Autodesk Fusion 360 part; units mm, degrees
(part 2 of 2)
sketch "Skizze17" plane through (0, 8, 0) normal (0, 1, 0) x (-1, 0, 0)
  spline S0 degree 3 poles (13.6382, 4.4313) (13.5302, 4.764) (13.3982, 5.084) (13.1091, 5.6313) (12.979, 5.7983) (12.7664, 6.018) (12.6585, 6.0998) (12.4173, 6.2178) (12.2929, 6.2453) (11.9322, 6.267) (11.6792, 6.209) (10.9713, 5.9696) (10.4381, 5.7266) (9.6899, 5.336) (9.4122, 5.1477) (9.0348, 4.7941) (8.8234, 4.5529) (8.5425, 3.9264) (8.498, 3.6504) (8.4775, 3.1972) (8.4959, 2.9778) (8.559, 2.7826) (8.5803, 2.717) (8.6261, 2.5931) (8.8115, 2.2891) (8.9377, 2.1162) (9.2854, 1.782) (9.4864, 1.6516) (10.0239, 1.4143) (10.3245, 1.381) (10.6864, 1.3735) (11.2116, 1.3812) (12.7231, 1.7144) (12.9818, 1.813) (13.2963, 1.9497) (13.4267, 2.0277) (13.6341, 2.2058) (13.7097, 2.3032) (13.8353, 2.5437) (13.8748, 2.6944) (13.921, 3.1631) (13.8758, 3.4676) (13.7815, 3.9466) (13.7161, 4.1922) (13.6382, 4.4313) knots -0.557189 -0.557189 -0.557189 -0.557189 -0.528825 -0.528825 -0.49746 -0.49746 -0.469449 -0.469449 -0.438886 -0.438886 -0.380684 -0.380684 -0.293014 -0.293014 -0.196609 -0.196609 -0.126355 -0.126355 -0.061556 -0.061556 0 0 0 0.020699 0.020699 0.037386 0.037386 0.056379 0.056379 0.086419 0.086419 0.099545 0.099545 0.108574 0.108574 0.118089 0.118089 0.127425 0.127425 0.139171 0.139171 0.160415 0.160415 0.180805 0.180805 0.180805 0.180805
  spline S1 degree 3 poles (8.4288, 11.6013) (8.146, 11.8071) (7.8511, 11.9884) (7.2955, 12.2611) (7.0921, 12.3198) (6.791, 12.3725) (6.6556, 12.3753) (6.391, 12.329) (6.2743, 12.2782) (5.9697, 12.0837) (5.7991, 11.8881) (5.3671, 11.2782) (5.0786, 10.7683) (4.7028, 10.0125) (4.5889, 9.6969) (4.4914, 9.189) (4.4621, 8.8696) (4.6031, 8.1977) (4.7294, 7.9482) (4.9792, 7.5696) (5.123, 7.4029) (5.2888, 7.2821) (5.3446, 7.2414) (5.4545, 7.1681) (5.7831, 7.0312) (5.9869, 6.9655) (6.4647, 6.8995) (6.7039, 6.9122) (7.2782, 7.0361) (7.5409, 7.1858) (7.8381, 7.3925) (8.2585, 7.7074) (9.2855, 8.8654) (9.4368, 9.0973) (9.6109, 9.3927) (9.6706, 9.5325) (9.7337, 9.7985) (9.7376, 9.9217) (9.6979, 10.1901) (9.6412, 10.3352) (9.4031, 10.7416) (9.1875, 10.9614) (8.8297, 11.2934) (8.6324, 11.4537) (8.4288, 11.6013) knots -0.557189 -0.557189 -0.557189 -0.557189 -0.528825 -0.528825 -0.49746 -0.49746 -0.469449 -0.469449 -0.438886 -0.438886 -0.380684 -0.380684 -0.293014 -0.293014 -0.196609 -0.196609 -0.126355 -0.126355 -0.061556 -0.061556 0 0 0 0.020699 0.020699 0.037386 0.037386 0.056379 0.056379 0.086419 0.086419 0.099545 0.099545 0.108574 0.108574 0.118089 0.118089 0.127425 0.127425 0.139171 0.139171 0.160415 0.160415 0.180805 0.180805 0.180805 0.180805
  spline S2 degree 3 poles (-13.6382, -4.4313) (-13.5302, -4.764) (-13.3982, -5.084) (-13.1091, -5.6313) (-12.979, -5.7983) (-12.7664, -6.018) (-12.6585, -6.0998) (-12.4173, -6.2178) (-12.2929, -6.2453) (-11.9322, -6.267) (-11.6792, -6.209) (-10.9713, -5.9696) (-10.4381, -5.7266) (-9.6899, -5.336) (-9.4122, -5.1477) (-9.0348, -4.7941) (-8.8234, -4.5529) (-8.5425, -3.9264) (-8.498, -3.6504) (-8.4775, -3.1972) (-8.4959, -2.9778) (-8.559, -2.7826) (-8.5803, -2.717) (-8.6261, -2.5931) (-8.8115, -2.2891) (-8.9377, -2.1162) (-9.2854, -1.782) (-9.4864, -1.6516) (-10.0239, -1.4143) (-10.3245, -1.381) (-10.6864, -1.3735) (-11.2116, -1.3812) (-12.7231, -1.7144) (-12.9818, -1.813) (-13.2963, -1.9497) (-13.4267, -2.0277) (-13.6341, -2.2058) (-13.7097, -2.3032) (-13.8353, -2.5437) (-13.8748, -2.6944) (-13.921, -3.1631) (-13.8758, -3.4676) (-13.7815, -3.9466) (-13.7161, -4.1922) (-13.6382, -4.4313) knots -0.557189 -0.557189 -0.557189 -0.557189 -0.528825 -0.528825 -0.49746 -0.49746 -0.469449 -0.469449 -0.438886 -0.438886 -0.380684 -0.380684 -0.293014 -0.293014 -0.196609 -0.196609 -0.126355 -0.126355 -0.061556 -0.061556 0 0 0 0.020699 0.020699 0.037386 0.037386 0.056379 0.056379 0.086419 0.086419 0.099545 0.099545 0.108574 0.108574 0.118089 0.118089 0.127425 0.127425 0.139171 0.139171 0.160415 0.160415 0.180805 0.180805 0.180805 0.180805
  spline S3 degree 3 poles (13.6382, -4.4313) (13.7464, -4.0987) (13.8277, -3.7622) (13.9155, -3.1495) (13.9084, -2.9379) (13.8655, -2.6353) (13.8263, -2.5057) (13.7005, -2.2684) (13.6161, -2.173) (13.337, -1.9434) (13.0982, -1.8416) (12.3848, -1.6193) (11.8106, -1.5025) (10.9757, -1.3786) (10.6404, -1.3678) (10.1272, -1.432) (9.8143, -1.5029) (9.2189, -1.8446) (9.0206, -2.0418) (8.7377, -2.3964) (8.6236, -2.5846) (8.56, -2.7797) (8.5386, -2.8453) (8.5028, -2.9724) (8.4741, -3.3273) (8.4746, -3.5414) (8.5595, -4.0162) (8.6455, -4.2398) (8.9408, -4.7477) (9.1644, -4.9513) (9.4528, -5.1701) (9.8822, -5.4726) (11.3009, -6.0915) (11.5681, -6.1637) (11.9029, -6.238) (12.0543, -6.2516) (12.3268, -6.2294) (12.4451, -6.195) (12.6881, -6.0743) (12.8087, -5.9756) (13.1216, -5.6236) (13.264, -5.3506) (13.4692, -4.9077) (13.5607, -4.6705) (13.6382, -4.4313) knots -0.557189 -0.557189 -0.557189 -0.557189 -0.528825 -0.528825 -0.49746 -0.49746 -0.469449 -0.469449 -0.438886 -0.438886 -0.380684 -0.380684 -0.293014 -0.293014 -0.196609 -0.196609 -0.126355 -0.126355 -0.061556 -0.061556 0 0 0 0.020699 0.020699 0.037386 0.037386 0.056379 0.056379 0.086419 0.086419 0.099545 0.099545 0.108574 0.108574 0.118089 0.118089 0.127425 0.127425 0.139171 0.139171 0.160415 0.160415 0.180805 0.180805 0.180805 0.180805
  spline S4 degree 3 poles (8.4288, -11.6013) (8.7119, -11.3959) (8.9755, -11.1714) (9.4066, -10.7273) (9.5253, -10.552) (9.6685, -10.2819) (9.7129, -10.154) (9.7506, -9.8881) (9.7384, -9.7613) (9.6475, -9.4116) (9.5142, -9.1888) (9.0677, -8.5896) (8.6718, -8.1576) (8.0692, -7.5667) (7.8043, -7.3609) (7.3514, -7.1111) (7.0566, -6.9846) (6.374, -6.9111) (6.0977, -6.954) (5.6604, -7.0746) (5.4575, -7.1598) (5.2913, -7.2802) (5.2354, -7.3207) (5.1318, -7.4026) (4.9, -7.6728) (4.7745, -7.8463) (4.5641, -8.2803) (4.5023, -8.5117) (4.4427, -9.0962) (4.5039, -9.3924) (4.6086, -9.7389) (4.7781, -10.2361) (5.5621, -11.5706) (5.7359, -11.7861) (5.963, -12.043) (6.0775, -12.143) (6.311, -12.2852) (6.427, -12.327) (6.6945, -12.3721) (6.8501, -12.3631) (7.3101, -12.2622) (7.5858, -12.1251) (8.0121, -11.8875) (8.2256, -11.7493) (8.4288, -11.6013) knots -0.557189 -0.557189 -0.557189 -0.557189 -0.528825 -0.528825 -0.49746 -0.49746 -0.469449 -0.469449 -0.438886 -0.438886 -0.380684 -0.380684 -0.293014 -0.293014 -0.196609 -0.196609 -0.126355 -0.126355 -0.061556 -0.061556 0 0 0 0.020699 0.020699 0.037386 0.037386 0.056379 0.056379 0.086419 0.086419 0.099545 0.099545 0.108574 0.108574 0.118089 0.118089 0.127425 0.127425 0.139171 0.139171 0.160415 0.160415 0.180805 0.180805 0.180805 0.180805
  spline S5 degree 3 poles (-8.4288, -11.6013) (-8.146, -11.8071) (-7.8511, -11.9884) (-7.2955, -12.2611) (-7.0921, -12.3198) (-6.791, -12.3725) (-6.6556, -12.3753) (-6.391, -12.329) (-6.2743, -12.2782) (-5.9697, -12.0837) (-5.7991, -11.8881) (-5.3671, -11.2782) (-5.0786, -10.7683) (-4.7028, -10.0125) (-4.5889, -9.6969) (-4.4914, -9.189) (-4.4621, -8.8696) (-4.6031, -8.1977) (-4.7294, -7.9482) (-4.9792, -7.5696) (-5.123, -7.4029) (-5.2888, -7.2821) (-5.3446, -7.2414) (-5.4545, -7.1681) (-5.7831, -7.0312) (-5.9869, -6.9655) (-6.4647, -6.8995) (-6.7039, -6.9122) (-7.2782, -7.0361) (-7.5409, -7.1858) (-7.8381, -7.3925) (-8.2585, -7.7074) (-9.2855, -8.8654) (-9.4368, -9.0973) (-9.6109, -9.3927) (-9.6706, -9.5325) (-9.7337, -9.7985) (-9.7376, -9.9217) (-9.6979, -10.1901) (-9.6412, -10.3352) (-9.4031, -10.7416) (-9.1875, -10.9614) (-8.8297, -11.2934) (-8.6324, -11.4537) (-8.4288, -11.6013) knots -0.557189 -0.557189 -0.557189 -0.557189 -0.528825 -0.528825 -0.49746 -0.49746 -0.469449 -0.469449 -0.438886 -0.438886 -0.380684 -0.380684 -0.293014 -0.293014 -0.196609 -0.196609 -0.126355 -0.126355 -0.061556 -0.061556 0 0 0 0.020699 0.020699 0.037386 0.037386 0.056379 0.056379 0.086419 0.086419 0.099545 0.099545 0.108574 0.108574 0.118089 0.118089 0.127425 0.127425 0.139171 0.139171 0.160415 0.160415 0.180805 0.180805 0.180805 0.180805
  spline S6 degree 3 poles (0, -14.34) (0.3498, -14.3402) (0.6949, -14.3135) (1.3047, -14.2077) (1.5038, -14.1356) (1.7784, -14.0012) (1.8895, -13.9239) (2.0763, -13.7309) (2.141, -13.6212) (2.2731, -13.2848) (2.2961, -13.0262) (2.2871, -12.279) (2.2207, -11.6968) (2.0805, -10.8645) (1.9872, -10.5423) (1.7676, -10.074) (1.6035, -9.7984) (1.0945, -9.3377) (0.8457, -9.2101) (0.421, -9.0506) (0.2067, -9.0002) (0.0015, -9) (-0.0675, -8.9999) (-0.1994, -9.0052) (-0.5458, -9.0876) (-0.7493, -9.1542) (-1.1746, -9.3816) (-1.3607, -9.5325) (-1.7524, -9.9703) (-1.877, -10.2459) (-1.996, -10.5878) (-2.151, -11.0897) (-2.3012, -12.6301) (-2.2873, -12.9067) (-2.2545, -13.248) (-2.2206, -13.3961) (-2.1153, -13.6485) (-2.0461, -13.7504) (-1.8562, -13.9442) (-1.725, -14.0283) (-1.2936, -14.2171) (-0.99, -14.2682) (-0.5053, -14.3266) (-0.2515, -14.3403) (0, -14.34) knots -0.557189 -0.557189 -0.557189 -0.557189 -0.528825 -0.528825 -0.49746 -0.49746 -0.469449 -0.469449 -0.438886 -0.438886 -0.380684 -0.380684 -0.293014 -0.293014 -0.196609 -0.196609 -0.126355 -0.126355 -0.061556 -0.061556 0 0 0 0.020699 0.020699 0.037386 0.037386 0.056379 0.056379 0.086419 0.086419 0.099545 0.099545 0.108574 0.108574 0.118089 0.118089 0.127425 0.127425 0.139171 0.139171 0.160415 0.160415 0.180805 0.180805 0.180805 0.180805
  spline S7 degree 3 poles (-13.6382, 4.4313) (-13.7464, 4.0987) (-13.8277, 3.7622) (-13.9155, 3.1495) (-13.9084, 2.9379) (-13.8655, 2.6353) (-13.8263, 2.5057) (-13.7005, 2.2684) (-13.6161, 2.173) (-13.337, 1.9434) (-13.0982, 1.8416) (-12.3848, 1.6193) (-11.8106, 1.5025) (-10.9757, 1.3786) (-10.6404, 1.3678) (-10.1272, 1.432) (-9.8143, 1.5029) (-9.2189, 1.8446) (-9.0206, 2.0418) (-8.7377, 2.3964) (-8.6236, 2.5846) (-8.56, 2.7797) (-8.5386, 2.8453) (-8.5028, 2.9724) (-8.4741, 3.3273) (-8.4746, 3.5414) (-8.5595, 4.0162) (-8.6455, 4.2398) (-8.9408, 4.7477) (-9.1644, 4.9513) (-9.4528, 5.1701) (-9.8822, 5.4726) (-11.3009, 6.0915) (-11.5681, 6.1637) (-11.9029, 6.238) (-12.0543, 6.2516) (-12.3268, 6.2294) (-12.4451, 6.195) (-12.6881, 6.0743) (-12.8087, 5.9756) (-13.1216, 5.6236) (-13.264, 5.3506) (-13.4692, 4.9077) (-13.5607, 4.6705) (-13.6382, 4.4313) knots -0.557189 -0.557189 -0.557189 -0.557189 -0.528825 -0.528825 -0.49746 -0.49746 -0.469449 -0.469449 -0.438886 -0.438886 -0.380684 -0.380684 -0.293014 -0.293014 -0.196609 -0.196609 -0.126355 -0.126355 -0.061556 -0.061556 0 0 0 0.020699 0.020699 0.037386 0.037386 0.056379 0.056379 0.086419 0.086419 0.099545 0.099545 0.108574 0.108574 0.118089 0.118089 0.127425 0.127425 0.139171 0.139171 0.160415 0.160415 0.180805 0.180805 0.180805 0.180805
  spline S8 degree 3 poles (-8.4288, 11.6013) (-8.7119, 11.3959) (-8.9755, 11.1714) (-9.4066, 10.7273) (-9.5253, 10.552) (-9.6685, 10.2819) (-9.7129, 10.154) (-9.7506, 9.8881) (-9.7384, 9.7613) (-9.6475, 9.4116) (-9.5142, 9.1888) (-9.0677, 8.5896) (-8.6718, 8.1576) (-8.0692, 7.5667) (-7.8043, 7.3609) (-7.3514, 7.1111) (-7.0566, 6.9846) (-6.374, 6.9111) (-6.0977, 6.954) (-5.6604, 7.0746) (-5.4575, 7.1598) (-5.2913, 7.2802) (-5.2354, 7.3207) (-5.1318, 7.4026) (-4.9, 7.6728) (-4.7745, 7.8463) (-4.5641, 8.2803) (-4.5023, 8.5117) (-4.4427, 9.0962) (-4.5039, 9.3924) (-4.6086, 9.7389) (-4.7781, 10.2361) (-5.5621, 11.5706) (-5.7359, 11.7861) (-5.963, 12.043) (-6.0775, 12.143) (-6.311, 12.2852) (-6.427, 12.327) (-6.6945, 12.3721) (-6.8501, 12.3631) (-7.3101, 12.2622) (-7.5858, 12.1251) (-8.0121, 11.8875) (-8.2256, 11.7493) (-8.4288, 11.6013) knots -0.557189 -0.557189 -0.557189 -0.557189 -0.528825 -0.528825 -0.49746 -0.49746 -0.469449 -0.469449 -0.438886 -0.438886 -0.380684 -0.380684 -0.293014 -0.293014 -0.196609 -0.196609 -0.126355 -0.126355 -0.061556 -0.061556 0 0 0 0.020699 0.020699 0.037386 0.037386 0.056379 0.056379 0.086419 0.086419 0.099545 0.099545 0.108574 0.108574 0.118089 0.118089 0.127425 0.127425 0.139171 0.139171 0.160415 0.160415 0.180805 0.180805 0.180805 0.180805
  spline S9 degree 3 poles (0, 14.34) (-0.3498, 14.3402) (-0.6949, 14.3135) (-1.3047, 14.2077) (-1.5038, 14.1356) (-1.7784, 14.0012) (-1.8895, 13.9239) (-2.0763, 13.7309) (-2.141, 13.6212) (-2.2731, 13.2848) (-2.2961, 13.0262) (-2.2871, 12.279) (-2.2207, 11.6968) (-2.0805, 10.8645) (-1.9872, 10.5423) (-1.7676, 10.074) (-1.6035, 9.7984) (-1.0945, 9.3377) (-0.8457, 9.2101) (-0.421, 9.0506) (-0.2067, 9.0002) (-0.0015, 9) (0.0675, 8.9999) (0.1994, 9.0052) (0.5458, 9.0876) (0.7493, 9.1542) (1.1746, 9.3816) (1.3607, 9.5325) (1.7524, 9.9703) (1.877, 10.2459) (1.996, 10.5878) (2.151, 11.0897) (2.3012, 12.6301) (2.2873, 12.9067) (2.2545, 13.248) (2.2206, 13.3961) (2.1153, 13.6485) (2.0461, 13.7504) (1.8562, 13.9442) (1.725, 14.0283) (1.2936, 14.2171) (0.99, 14.2682) (0.5053, 14.3266) (0.2515, 14.3403) (0, 14.34) knots -0.557189 -0.557189 -0.557189 -0.557189 -0.528825 -0.528825 -0.49746 -0.49746 -0.469449 -0.469449 -0.438886 -0.438886 -0.380684 -0.380684 -0.293014 -0.293014 -0.196609 -0.196609 -0.126355 -0.126355 -0.061556 -0.061556 0 0 0 0.020699 0.020699 0.037386 0.037386 0.056379 0.056379 0.086419 0.086419 0.099545 0.099545 0.108574 0.108574 0.118089 0.118089 0.127425 0.127425 0.139171 0.139171 0.160415 0.160415 0.180805 0.180805 0.180805 0.180805
  circle A0 centre (0, 0) radius 16.0986
  circle A1 centre (0, 0) radius 3.5
  line L0 (3.7528, -6.5) -> (7.5056, 0)
  line L1 (7.5056, 0) -> (3.7528, 6.5)
  line L2 (3.7528, 6.5) -> (-3.7528, 6.5)
  line L3 (-3.7528, 6.5) -> (-7.5056, 0)
  line L4 (-7.5056, 0) -> (-3.7528, -6.5)
  line L5 (-3.7528, -6.5) -> (3.7528, -6.5)
  circle A2 centre (0, 0) radius 20.6725
  dimension "d112" = 7
  dimension "d113" = 13
  measures "d112" diameter of A1
  measures "d113" distance of L1 L4
extrude "Extrusion17" cut sketch "Skizze17" against normal blind 3 contours A1 | L0 L1 L2 L3 L4 L5 bodies 1
extrude "Extrusion18" cut sketch "Skizze17" against normal through all contours A1 bodies 1
sketch "Skizze18" plane through (0, -1, 0) normal (0, -1, 0) x (1, 0, 0)
  circle A0 centre (0, 0) radius 3.5
  circle A1 centre (0, 0) radius 20.6725
  circle A2 centre (0, 0) radius 20.6725
  circle A3 centre (0, 0) radius 20.1725
  dimension "d117" = 0.5
  measures "d117" distance of A1 A3
extrude "Extrusion19" cut sketch "Skizze18" against normal through all contours A1 A2 bodies 1
sketch "Sketch19" plane through (0, 8, 0) normal (0, 1, 0) x (-1, 0, 0)
  circle A0 centre (0, 0) radius 20.1725
  line L0 (7.5056, 0) -> (3.7528, -6.5)
  line L1 (3.7528, -6.5) -> (-3.7528, -6.5)
  line L2 (-3.7528, -6.5) -> (-7.5056, 0)
  line L3 (-7.5056, 0) -> (-3.7528, 6.5)
  line L4 (-3.7528, 6.5) -> (3.7528, 6.5)
  line L5 (3.7528, 6.5) -> (7.5056, 0)
  line L6 (0, 0) -> (0, -12)
  dimension "d125" = 12
  measures "d125" distance of A0.centre
hole "Hole1" at (0, 8, -12) direction (0, -1, 0) diameter 4.2 depth 20 tip angle 118 counterbore diameter 7.2 counterbore depth 4.2 bodies 1
pattern_circular "C-Pattern4" count 4 over 360 about axis through (0, 1.75, 0) along (0, 1, 0) of "Hole1"
equation "d8 = PLD"
equation "teethCount = 42"
equation "PLD = 0.381 mm"
equation "outerDiameter = ( ( pitchLength * teethCount ) / PI ) - ( 2 * PLD )"
equation "pitchLength = 3 mm"
equation "pitchDiameter = ( pitchLength * teethCount ) / PI"
equation "anglePerTooth = 360 deg / teethCount"
equation "d19 = anglePerTooth / 2"
equation "d23 = outerDiameter / 2"
equation "d25 = beltWidth"
equation "d28 = teethCount"
equation "d30 = outerDiameter + 2 mm"
equation "d33 = outerDiameter + 2 mm"
equation "beltWidth = 7 mm"
equation "magicSplintOffset = 10 mm"
equation "magicAxelFactor = 0.5"
equation "holeOffsetToPD = 3 mm"
equation "holeCount = 10"
equation "holeInnerDiameter = 18 mm"
equation "holeToFillRatio = 0.6"
